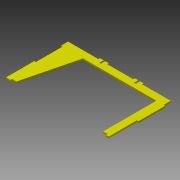
# Autodesk Inventor part: frontLeg
Saved by Autodesk Inventor 2015 SP1 (Build 190203100, 203)
## iProperties
Created: 2015-04-09
Part Number: frontLeg
Material: Generic
Document SubType Name: Modeling
Designer: Iain
Density: 1 g/cm^3
Appearance: Smooth - Yellow
Author: Iain
Autodesk Inventor part; units mm, degrees
sketch "Sketch1" plane through (0, 0, 0) normal (0, 0, 1) x (1, 0, 0)
  line L0 (-590, 351) -> (590, 351)
  line L1 (590, 351) -> (590, -351)
  line L2 (590, -351) -> (-590, -351)
  line L3 (-590, -351) -> (-590, 351)
  point P0 (0, 0)
  point P1 (590, 0)
  point P2 (0, 351)
  dimension "d0" = 1180
  dimension "d1" = 702
  constraints: 8 end point, 2 midpoint, 2 parallel, 1 horizontal, 1 horizontal alignment, 1 perpendicular, 1 vertical alignment
  measures "d0" distance of L0.start L0.end
  measures "d1" distance of L2.end L0.start
extrude "Extrusion1" add sketch "Sketch1" along normal blind 18
sketch "Sketch2" plane through (0, 0, 18) normal (0, 0, 1) x (1, 0, 0)
  line L0 (590, 351) -> (-590, 351) projected
  line L1 (-590, 351) -> (-590, -351) projected
  line L2 (-590, -351) -> (590, -351) projected
  line L3 (590, -351) -> (590, 351) projected
  line L4 (-590, -351) -> (-490, -351) construction
  line L5 (-590, 351) -> (-590, -351) construction
  line L6 (590, 351) -> (-590, 351) construction
  line L7 (0, 351) -> (0, -351) construction
  line L8 (590, -351) -> (490, -351) construction
  line L9 (-590, 271) -> (590, 271) construction
  line L10 (-590, 271) -> (-340, 271) construction
  line L11 (-340, 271) -> (490, 271)
  line L12 (490, 271) -> (490, -351)
  line L13 (490, -351) -> (-490, -351)
  line L14 (-490, -351) -> (-490, -333)
  line L15 (-490, -333) -> (-340, 271)
  point P0 (0, 0)
  point P1 (-590, 0)
  point P2 (-590, 0)
  point P3 (-540, -351)
  point P4 (540, -351)
  point P5 (-590, 0)
  point P6 (590, 0)
  point P7 (-590, 0)
  point P8 (-465, 271)
  point P9 (0, 271)
  dimension "d4" = 100
  dimension "d5" = 80
  dimension "d6" = 250
  dimension "d97" = 18
  constraints: 20 end point, 10 midpoint, 4 symmetric about line, 4 vertical alignment, 3 horizontal, 3 perpendicular, 2 horizontal alignment, 1 collinear, 1 point on line
  measures "d4" distance of L4.start L4.end
  measures "d5" distance between parallel lines of L0 L9
  measures "d6" distance of L10.start L10.end
  measures "d97" distance of L4.end L14.end
extrude "Extrusion2" cut sketch "Sketch2" against normal blind 18 contours L2 L14 L15 L11 L12
sketch "Sketch3" plane through (0, 0, 18) normal (0, 0, 1) x (1, 0, 0)
  line L0 (-340, 271) -> (490, 271) projected
  line L1 (490, 271) -> (490, -351) projected
  line L2 (490, -351) -> (590, -351) projected
  line L3 (590, -351) -> (590, 351) projected
  line L4 (590, 351) -> (-590, 351) projected
  line L5 (-590, 351) -> (-590, -351) projected
  line L6 (-540, -333) -> (540, -333)
  line L7 (540, -333) -> (540, -351)
  line L8 (540, -351) -> (-540, -351)
  line L9 (-540, -351) -> (-540, -333)
  line L10 (490, -351) -> (590, -351) projected
  line L11 (-590, -351) -> (590, -351) projected
  line L12 (-590, -351) -> (-490, -351) projected
  line L13 (-490, -351) -> (-490, -333) projected
  line L14 (-490, -333) -> (-340, 271) projected
  point P0 (0, 0)
  point P1 (540, -351)
  point P2 (0, -351)
  point P3 (-540, -351)
  point P4 (540, -342)
  point P5 (540, -351)
  point P6 (-540, -342)
  point P7 (-540, -351)
  dimension "d10" = 18
  constraints: 8 end point, 5 midpoint, 2 parallel, 2 vertical alignment, 1 horizontal, 1 horizontal alignment, 1 perpendicular, 1 point on line
  measures "d10" distance of L6.end L7.end
extrude "Extrusion3" cut sketch "Sketch3" against normal blind 18 contours L13 L8 L9 L6 | L6 L1 L8 L13 | L6 L7 L2 L1
sketch "Sketch4" plane through (0, 0, 18) normal (0, 0, 1) x (1, 0, 0)
  line L0 (540, -333) -> (540, -351) projected
  line L1 (540, -351) -> (590, -351) projected
  line L2 (590, -351) -> (590, 351) projected
  line L3 (590, 351) -> (-590, 351) projected
  line L4 (-590, 351) -> (-590, -351) projected
  line L5 (-590, -351) -> (-540, -351) projected
  line L6 (-540, -351) -> (-540, -333) projected
  line L7 (-540, -333) -> (-490, -333) projected
  line L8 (-340, 271) -> (490, 271) projected
  line L9 (490, 271) -> (490, -333) projected
  line L10 (490, -333) -> (540, -333) projected
  line L11 (590, -31) -> (572, -31)
  line L12 (572, -31) -> (572, -351)
  line L13 (572, -351) -> (590, -351)
  line L14 (590, -351) -> (590, -31)
  line L15 (-490, -333) -> (-340, 271) projected
  point P0 (0, 0)
  point P1 (581, -351)
  point P2 (565, -351)
  point P3 (590, -191)
  point P4 (590, 0)
  point P5 (581, -31)
  point P6 (490, -31)
  dimension "d13" = 18
  constraints: 8 end point, 6 midpoint, 2 horizontal alignment, 2 parallel, 1 horizontal, 1 perpendicular, 1 vertical alignment
  measures "d13" distance of L11.start L11.end
extrude "Extrusion4" cut sketch "Sketch4" against normal blind 18 contours L12 L11 L2 L1
sketch "Sketch5" plane through (0, 0, 18) normal (0, 0, 1) x (1, 0, 0)
  line L0 (-590, 271) -> (-572, 271)
  line L1 (-572, 271) -> (-572, -31)
  line L2 (-572, -31) -> (-590, -31)
  line L3 (-590, -31) -> (-590, 271)
  line L4 (572, -31) -> (590, -31) projected
  line L5 (590, -31) -> (590, 351) projected
  line L6 (590, 351) -> (-590, 351) projected
  line L7 (-590, 351) -> (-590, -351) projected
  line L8 (-590, -351) -> (-540, -351) projected
  line L9 (-540, -351) -> (-540, -333) projected
  line L10 (-540, -333) -> (-490, -333) projected
  line L11 (-340, 271) -> (490, 271) projected
  line L12 (490, 271) -> (490, -333) projected
  line L13 (490, -333) -> (540, -333) projected
  line L14 (540, -333) -> (540, -351) projected
  line L15 (540, -351) -> (572, -351) projected
  line L16 (572, -351) -> (572, -31) projected
  line L17 (-490, -333) -> (-340, 271) projected
  point P0 (0, 0)
  point P1 (-581, -31)
  point P2 (581, -31)
  point P3 (-581, 271)
  point P4 (75, 271)
  point P5 (-590, 120)
  point P6 (-590, 0)
  dimension "d16" = 18
  constraints: 8 end point, 6 midpoint, 2 horizontal alignment, 2 parallel, 1 horizontal, 1 perpendicular, 1 vertical alignment
  measures "d16" distance of L0.start L0.end
extrude "Extrusion5" cut sketch "Sketch5" against normal blind 18 contours L0 L1 L2 L3
sketch "Sketch6" plane through (0, 0, 18) normal (0, 0, 1) x (1, 0, 0)
  line L0 (-590, 271) -> (-572, 271) projected
  line L1 (-572, 271) -> (-572, -31) projected
  line L2 (-572, -31) -> (-590, -31) projected
  line L3 (-590, -31) -> (-590, -351) projected
  line L4 (-590, -351) -> (-540, -351) projected
  line L5 (-540, -351) -> (-540, -333) projected
  line L6 (-540, -333) -> (-490, -333) projected
  line L7 (-340, 271) -> (490, 271) projected
  line L8 (490, 271) -> (490, -333) projected
  line L9 (490, -333) -> (540, -333) projected
  line L10 (540, -333) -> (540, -351) projected
  line L11 (540, -351) -> (572, -351) projected
  line L12 (572, -351) -> (572, -31) projected
  line L13 (572, -31) -> (590, -31) projected
  line L14 (590, -31) -> (590, 351) projected
  line L15 (590, 351) -> (-590, 351) projected
  line L16 (-590, 351) -> (-590, 271) projected
  line L17 (590, 351) -> (572, 351)
  line L18 (572, 351) -> (572, 271)
  line L19 (572, 271) -> (590, 271)
  line L20 (590, 271) -> (590, 351)
  line L21 (-490, -333) -> (-340, 271) projected
  point P0 (0, 0)
  point P1 (581, 351)
  point P2 (0, 351)
  point P3 (581, 271)
  point P4 (75, 271)
  point P5 (590, 311)
  point P6 (590, 160)
  dimension "d19" = 18
  constraints: 8 end point, 6 midpoint, 2 horizontal alignment, 2 parallel, 1 horizontal, 1 perpendicular, 1 vertical alignment
  measures "d19" distance of L17.start L17.end
extrude "Extrusion6" cut sketch "Sketch6" against normal blind 18 contours L15 L14 L19 L18
fillet "Fillet1" radius 3.175 2 edges at (-340, 271, 9) (490, 271, 9)
sketch "Sketch7" plane through (0, 0, 18) normal (0, 0, 1) x (1, 0, 0)
  line L0 (-246.6667, 369) -> (-146.6667, 369)
  line L1 (-146.6667, 369) -> (-146.6667, 351)
  line L2 (-146.6667, 351) -> (-246.6667, 351)
  line L3 (-246.6667, 351) -> (-246.6667, 369)
  line L4 (590, 271) -> (572, 271) projected
  line L5 (572, 271) -> (572, 351) projected
  line L6 (572, 351) -> (-590, 351) projected
  line L7 (-590, 351) -> (-590, 271) projected
  line L8 (-590, 271) -> (-572, 271) projected
  line L9 (-572, 271) -> (-572, -31) projected
  line L10 (-572, -31) -> (-590, -31) projected
  line L11 (-590, -31) -> (-590, -351) projected
  line L12 (-590, -351) -> (-540, -351) projected
  line L13 (-540, -351) -> (-540, -333) projected
  line L14 (-540, -333) -> (-490, -333) projected
  arc A0 (-337.517, 271) -> (-340.5984, 268.5902) centre (-337.517, 267.825) ccw projected
  line L15 (-337.517, 271) -> (486.825, 271) projected
  arc A1 (490, 267.825) -> (486.825, 271) centre (486.825, 267.825) ccw projected
  line L16 (490, 267.825) -> (490, -333) projected
  line L17 (490, -333) -> (540, -333) projected
  line L18 (540, -333) -> (540, -351) projected
  line L19 (540, -351) -> (572, -351) projected
  line L20 (572, -351) -> (572, -31) projected
  line L21 (572, -31) -> (590, -31) projected
  line L22 (590, -31) -> (590, 271) projected
  line L23 (-490, -333) -> (-340.5984, 268.5902) projected
  point P0 (0, 0)
  point P1 (-196.6667, 351)
  point P2 (-9, 351)
  dimension "d23" = 18
  dimension "d24" = 100
  dimension "d25" = 393.3333
  constraints: 8 end point, 2 midpoint, 2 parallel, 1 horizontal, 1 horizontal alignment, 1 perpendicular
  measures "d23" distance of L0.end L1.end
  measures "d24" distance of L0.start L0.end
  measures "d25" distance of L6.end point (-196.667, 351)
extrude "Extrusion7" add sketch "Sketch7" against normal blind 18 contours L0 L1 L2 L3
ref_plane "Work Plane1" through (0, 351, 0) normal (-1, 0, 0) x (0, 0, 1)
mirror "Mirror1" about plane through (0, 351, 0) normal (-1, 0, 0) of "Extrusion7"
sketch "Sketch8" plane through (0, 0, 18) normal (0, 0, 1) x (1, 0, 0)
  line L0 (590, 271) -> (572, 271) projected
  line L1 (572, 271) -> (572, 351) projected
  line L2 (572, 351) -> (246.6667, 351) projected
  line L3 (246.6667, 351) -> (246.6667, 369) projected
  line L4 (246.6667, 369) -> (146.6667, 369) projected
  line L5 (146.6667, 369) -> (146.6667, 351) projected
  line L6 (146.6667, 351) -> (-146.6667, 351) projected
  line L7 (-146.6667, 369) -> (-146.6667, 351) projected
  line L8 (-246.6667, 369) -> (-146.6667, 369) projected
  line L9 (-246.6667, 351) -> (-246.6667, 369) projected
  line L10 (-246.6667, 351) -> (-590, 351) projected
  line L11 (-590, 351) -> (-590, 271) projected
  line L12 (-590, 271) -> (-572, 271) projected
  line L13 (-572, 271) -> (-572, -31) projected
  line L14 (-572, -31) -> (-590, -31) projected
  line L15 (-590, -31) -> (-590, -351) projected
  line L16 (-590, -351) -> (-540, -351) projected
  line L17 (-540, -351) -> (-540, -333) projected
  line L18 (-540, -333) -> (-490, -333) projected
  arc A0 (-337.517, 271) -> (-340.5984, 268.5902) centre (-337.517, 267.825) ccw projected
  line L19 (-337.517, 271) -> (486.825, 271) projected
  arc A1 (490, 267.825) -> (486.825, 271) centre (486.825, 267.825) ccw projected
  line L20 (490, 267.825) -> (490, -333) projected
  line L21 (490, -333) -> (540, -333) projected
  line L22 (540, -333) -> (540, -351) projected
  line L23 (540, -351) -> (572, -351) projected
  line L24 (572, -351) -> (572, -31) projected
  line L25 (572, -31) -> (590, -31) projected
  line L26 (590, -31) -> (590, 271) projected
  line L27 (-205.6667, 369) -> (-187.6667, 369)
  line L28 (-187.6667, 369) -> (-187.6667, 320)
  line L29 (-187.6667, 320) -> (-205.6667, 320)
  line L30 (-205.6667, 320) -> (-205.6667, 369)
  line L31 (-246.6667, 369) -> (-146.6667, 369) projected
  line L32 (486.825, 271) -> (-337.517, 271) construction
  line L33 (-490, -333) -> (-340.5984, 268.5902) projected
  point P0 (0, 0)
  point P1 (-196.6667, 369)
  point P2 (-196.6667, 369)
  point P3 (-196.6667, 369)
  point P4 (-196.6667, 320)
  point P5 (-590, 311)
  point P6 (-246.6667, 320)
  dimension "d28" = 18
  dimension "d31" = 49
  constraints: 8 end point, 5 midpoint, 2 coincident, 2 parallel, 1 horizontal, 1 horizontal alignment, 1 perpendicular
  measures "d28" distance of L27.start L27.end
  measures "d31" distance of L27.end L28.end
extrude "Extrusion8" cut sketch "Sketch8" against normal blind 18 contours L28 L29 L30 L8
mirror "Mirror2" about plane through (0, 351, 0) normal (-1, 0, 0) of "Extrusion8"
sketch "Sketch9" plane through (0, 0, 18) normal (0, 0, 1) x (1, 0, 0)
  line L0 (187.6667, 320) -> (187.6667, 369) projected
  line L1 (187.6667, 369) -> (146.6667, 369) projected
  line L2 (146.6667, 369) -> (146.6667, 351) projected
  line L3 (146.6667, 351) -> (-146.6667, 351) projected
  line L4 (-146.6667, 369) -> (-146.6667, 351) projected
  line L5 (-187.6667, 369) -> (-146.6667, 369) projected
  line L6 (-187.6667, 369) -> (-187.6667, 320) projected
  line L7 (-187.6667, 320) -> (-205.6667, 320) projected
  line L8 (-205.6667, 320) -> (-205.6667, 369) projected
  line L9 (-246.6667, 369) -> (-205.6667, 369) projected
  line L10 (-246.6667, 351) -> (-246.6667, 369) projected
  line L11 (-246.6667, 351) -> (-590, 351) projected
  line L12 (-590, 351) -> (-590, 271) projected
  line L13 (-590, 271) -> (-572, 271) projected
  line L14 (-572, 271) -> (-572, -31) projected
  line L15 (-572, -31) -> (-590, -31) projected
  line L16 (-590, -31) -> (-590, -351) projected
  line L17 (-590, -351) -> (-540, -351) projected
  line L18 (-540, -351) -> (-540, -333) projected
  line L19 (-540, -333) -> (-490, -333) projected
  arc A0 (-337.517, 271) -> (-340.5984, 268.5902) centre (-337.517, 267.825) ccw projected
  line L20 (-337.517, 271) -> (486.825, 271) projected
  arc A1 (490, 267.825) -> (486.825, 271) centre (486.825, 267.825) ccw projected
  line L21 (490, 267.825) -> (490, -333) projected
  line L22 (490, -333) -> (540, -333) projected
  line L23 (540, -333) -> (540, -351) projected
  line L24 (540, -351) -> (572, -351) projected
  line L25 (572, -351) -> (572, -31) projected
  line L26 (572, -31) -> (590, -31) projected
  line L27 (590, -31) -> (590, 271) projected
  line L28 (590, 271) -> (572, 271) projected
  line L29 (572, 271) -> (572, 351) projected
  line L30 (572, 351) -> (246.6667, 351) projected
  line L31 (246.6667, 351) -> (246.6667, 369) projected
  line L32 (246.6667, 369) -> (205.6667, 369) projected
  line L33 (205.6667, 369) -> (205.6667, 320) projected
  line L34 (205.6667, 320) -> (187.6667, 320) projected
  line L35 (-490, -333) -> (-340.5984, 268.5902) projected
  point P0 (0, 0)
  point P1 (-581, 311)
  point P2 (-590, 311)
  dimension "d32" = 9
  constraints: 1 horizontal alignment, 1 midpoint
  measures "d32" distance of point (-590, 311) point (-581, 311)
hole "Hole1" at (-581, 311, 18) direction (0, 0, -1) diameter 6.35 end through all
sketch "Sketch10" plane through (0, 0, 18) normal (0, 0, 1) x (1, 0, 0)
  circle A0 centre (-581, 311) radius 3.175 projected
  line L0 (187.6667, 320) -> (187.6667, 369) projected
  line L1 (187.6667, 369) -> (146.6667, 369) projected
  line L2 (146.6667, 369) -> (146.6667, 351) projected
  line L3 (146.6667, 351) -> (-146.6667, 351) projected
  line L4 (-146.6667, 369) -> (-146.6667, 351) projected
  line L5 (-187.6667, 369) -> (-146.6667, 369) projected
  line L6 (-187.6667, 369) -> (-187.6667, 320) projected
  line L7 (-187.6667, 320) -> (-205.6667, 320) projected
  line L8 (-205.6667, 320) -> (-205.6667, 369) projected
  line L9 (-246.6667, 369) -> (-205.6667, 369) projected
  line L10 (-246.6667, 351) -> (-246.6667, 369) projected
  line L11 (-246.6667, 351) -> (-590, 351) projected
  line L12 (-590, 351) -> (-590, 271) projected
  line L13 (-590, 271) -> (-572, 271) projected
  line L14 (-572, 271) -> (-572, -31) projected
  line L15 (-572, -31) -> (-590, -31) projected
  line L16 (-590, -31) -> (-590, -351) projected
  line L17 (-590, -351) -> (-540, -351) projected
  line L18 (-540, -351) -> (-540, -333) projected
  line L19 (-540, -333) -> (-490, -333) projected
  arc A1 (-337.517, 271) -> (-340.5984, 268.5902) centre (-337.517, 267.825) ccw projected
  line L20 (-337.517, 271) -> (486.825, 271) projected
  arc A2 (490, 267.825) -> (486.825, 271) centre (486.825, 267.825) ccw projected
  line L21 (490, 267.825) -> (490, -333) projected
  line L22 (490, -333) -> (540, -333) projected
  line L23 (540, -333) -> (540, -351) projected
  line L24 (540, -351) -> (572, -351) projected
  line L25 (572, -351) -> (572, -31) projected
  line L26 (572, -31) -> (590, -31) projected
  line L27 (590, -31) -> (590, 271) projected
  line L28 (590, 271) -> (572, 271) projected
  line L29 (572, 271) -> (572, 351) projected
  line L30 (572, 351) -> (246.6667, 351) projected
  line L31 (246.6667, 351) -> (246.6667, 369) projected
  line L32 (246.6667, 369) -> (205.6667, 369) projected
  line L33 (205.6667, 369) -> (205.6667, 320) projected
  line L34 (205.6667, 320) -> (187.6667, 320) projected
  line L35 (-581, -31) -> (-581, -333) construction
  line L36 (-490, -333) -> (-340.5984, 268.5902) projected
  point P0 (0, 0)
  point P1 (-581, -31)
  point P2 (-515, -333)
  point P3 (-581, -182)
  dimension "d40" = 9
  constraints: 3 midpoint, 2 end point, 1 coincident, 1 horizontal alignment, 1 vertical
  measures "d40" distance of L15.end L35.start
hole "Hole2" at (-581, -182, 18) direction (0, 0, -1) diameter 6.35 end through all
sketch "Sketch11" plane through (0, 0, 18) normal (0, 0, 1) x (1, 0, 0)
  circle A0 centre (-581, -182) radius 3.175 projected
  circle A1 centre (-581, 311) radius 3.175 projected
  line L0 (187.6667, 320) -> (187.6667, 369) projected
  line L1 (187.6667, 369) -> (146.6667, 369) projected
  line L2 (146.6667, 369) -> (146.6667, 351) projected
  line L3 (146.6667, 351) -> (-146.6667, 351) projected
  line L4 (-146.6667, 369) -> (-146.6667, 351) projected
  line L5 (-187.6667, 369) -> (-146.6667, 369) projected
  line L6 (-187.6667, 369) -> (-187.6667, 320) projected
  line L7 (-187.6667, 320) -> (-205.6667, 320) projected
  line L8 (-205.6667, 320) -> (-205.6667, 369) projected
  line L9 (-246.6667, 369) -> (-205.6667, 369) projected
  line L10 (-246.6667, 351) -> (-246.6667, 369) projected
  line L11 (-246.6667, 351) -> (-590, 351) projected
  line L12 (-590, 351) -> (-590, 271) projected
  line L13 (-590, 271) -> (-572, 271) projected
  line L14 (-572, 271) -> (-572, -31) projected
  line L15 (-572, -31) -> (-590, -31) projected
  line L16 (-590, -31) -> (-590, -351) projected
  line L17 (-590, -351) -> (-540, -351) projected
  line L18 (-540, -351) -> (-540, -333) projected
  line L19 (-540, -333) -> (-490, -333) projected
  arc A2 (-337.517, 271) -> (-340.5984, 268.5902) centre (-337.517, 267.825) ccw projected
  line L20 (-337.517, 271) -> (486.825, 271) projected
  arc A3 (490, 267.825) -> (486.825, 271) centre (486.825, 267.825) ccw projected
  line L21 (490, 267.825) -> (490, -333) projected
  line L22 (490, -333) -> (540, -333) projected
  line L23 (540, -333) -> (540, -351) projected
  line L24 (540, -351) -> (572, -351) projected
  line L25 (572, -351) -> (572, -31) projected
  line L26 (572, -31) -> (590, -31) projected
  line L27 (590, -31) -> (590, 271) projected
  line L28 (590, 271) -> (572, 271) projected
  line L29 (572, 271) -> (572, 351) projected
  line L30 (572, 351) -> (246.6667, 351) projected
  line L31 (246.6667, 351) -> (246.6667, 369) projected
  line L32 (246.6667, 369) -> (205.6667, 369) projected
  line L33 (205.6667, 369) -> (205.6667, 320) projected
  line L34 (205.6667, 320) -> (187.6667, 320) projected
  line L35 (-490, -333) -> (-340.5984, 268.5902) projected
  point P0 (0, 0)
  point P1 (581, 120)
  point P2 (590, 120)
  dimension "d48" = 9
  constraints: 1 horizontal alignment, 1 midpoint
  measures "d48" distance of point (590, 120) point (581, 120)
hole "Hole3" at (581, 120, 18) direction (0, 0, -1) diameter 6.35 end through all
sketch "Sketch12" plane through (0, 0, 18) normal (0, 0, 1) x (1, 0, 0)
  circle A0 centre (581, 120) radius 3.175 projected
  circle A1 centre (-581, -182) radius 3.175 projected
  circle A2 centre (-581, 311) radius 3.175 projected
  line L0 (187.6667, 320) -> (187.6667, 369) projected
  line L1 (187.6667, 369) -> (146.6667, 369) projected
  line L2 (146.6667, 369) -> (146.6667, 351) projected
  line L3 (146.6667, 351) -> (-146.6667, 351) projected
  line L4 (-146.6667, 369) -> (-146.6667, 351) projected
  line L5 (-187.6667, 369) -> (-146.6667, 369) projected
  line L6 (-187.6667, 369) -> (-187.6667, 320) projected
  line L7 (-187.6667, 320) -> (-205.6667, 320) projected
  line L8 (-205.6667, 320) -> (-205.6667, 369) projected
  line L9 (-246.6667, 369) -> (-205.6667, 369) projected
  line L10 (-246.6667, 351) -> (-246.6667, 369) projected
  line L11 (-246.6667, 351) -> (-590, 351) projected
  line L12 (-590, 351) -> (-590, 271) projected
  line L13 (-590, 271) -> (-572, 271) projected
  line L14 (-572, 271) -> (-572, -31) projected
  line L15 (-572, -31) -> (-590, -31) projected
  line L16 (-590, -31) -> (-590, -351) projected
  line L17 (-590, -351) -> (-540, -351) projected
  line L18 (-540, -351) -> (-540, -333) projected
  line L19 (-540, -333) -> (-490, -333) projected
  arc A3 (-337.517, 271) -> (-340.5984, 268.5902) centre (-337.517, 267.825) ccw projected
  line L20 (-337.517, 271) -> (486.825, 271) projected
  arc A4 (490, 267.825) -> (486.825, 271) centre (486.825, 267.825) ccw projected
  line L21 (490, 267.825) -> (490, -333) projected
  line L22 (490, -333) -> (540, -333) projected
  line L23 (540, -333) -> (540, -351) projected
  line L24 (540, -351) -> (572, -351) projected
  line L25 (572, -351) -> (572, -31) projected
  line L26 (572, -31) -> (590, -31) projected
  line L27 (590, -31) -> (590, 271) projected
  line L28 (590, 271) -> (572, 271) projected
  line L29 (572, 271) -> (572, 351) projected
  line L30 (572, 351) -> (246.6667, 351) projected
  line L31 (246.6667, 351) -> (246.6667, 369) projected
  line L32 (246.6667, 369) -> (205.6667, 369) projected
  line L33 (205.6667, 369) -> (205.6667, 320) projected
  line L34 (205.6667, 320) -> (187.6667, 320) projected
  line L35 (-196.6667, 320) -> (-196.6667, 271) construction
  line L36 (-187.6667, 320) -> (-205.6667, 320) construction
  line L37 (-490, -333) -> (-340.5984, 268.5902) projected
  point P0 (0, 0)
  point P1 (74.654, 271)
  point P2 (-196.6667, 295.5)
  point P3 (-196.6667, 295.5)
  constraints: 4 midpoint, 2 coincident, 2 end point, 1 horizontal alignment, 1 vertical, 1 vertical alignment
hole "Hole4" at (-196.6667, 295.5, 18) direction (0, 0, -1) diameter 6.35 end through all
mirror "Mirror3" about plane through (0, 351, 0) normal (-1, 0, 0) of "Hole4"
sketch "Sketch13" plane through (0, 0, 18) normal (0, 0, 1) x (1, 0, 0)
  line L0 (-590, 271) -> (-572, 271) projected
  point P0 (0, 0)
  point P1 (-572, 267.825)
  dimension "d63" = 3.175
  constraints: 1 vertical alignment
  measures "d63" distance from line of L0 point (-572, 267.825)
hole "Hole5" at (-572, 267.825, 18) direction (0, 0, -1) diameter 6.35 end through all
ref_plane "Work Plane2" through (-590, 120, 0) normal (0, -1, 0) x (1, 0, 0)
mirror "Mirror4" about plane through (-590, 120, 0) normal (0, -1, 0) of "Hole5"
sketch "Sketch14" plane through (0, 0, 18) normal (0, 0, 1) x (1, 0, 0)
  arc A0 (-572, -31) -> (-572, -24.65) centre (-572, -27.825) ccw projected
  line L0 (-572, -31) -> (-590, -31) projected
  line L1 (-590, -31) -> (-590, -351) projected
  line L2 (-590, -351) -> (-540, -351) projected
  line L3 (-540, -351) -> (-540, -333) projected
  line L4 (-540, -333) -> (-490, -333) projected
  arc A1 (-337.517, 271) -> (-340.5984, 268.5902) centre (-337.517, 267.825) ccw projected
  line L5 (-337.517, 271) -> (486.825, 271) projected
  arc A2 (490, 267.825) -> (486.825, 271) centre (486.825, 267.825) ccw projected
  line L6 (490, 267.825) -> (490, -333) projected
  line L7 (490, -333) -> (540, -333) projected
  line L8 (540, -333) -> (540, -351) projected
  line L9 (540, -351) -> (572, -351) projected
  line L10 (572, -351) -> (572, -31) projected
  line L11 (572, -31) -> (590, -31) projected
  line L12 (590, -31) -> (590, 271) projected
  line L13 (590, 271) -> (572, 271) projected
  line L14 (572, 271) -> (572, 351) projected
  line L15 (572, 351) -> (246.6667, 351) projected
  line L16 (246.6667, 351) -> (246.6667, 369) projected
  line L17 (246.6667, 369) -> (205.6667, 369) projected
  line L18 (205.6667, 369) -> (205.6667, 320) projected
  line L19 (205.6667, 320) -> (187.6667, 320) projected
  line L20 (187.6667, 320) -> (187.6667, 369) projected
  line L21 (187.6667, 369) -> (146.6667, 369) projected
  line L22 (146.6667, 369) -> (146.6667, 351) projected
  line L23 (146.6667, 351) -> (-146.6667, 351) projected
  line L24 (-146.6667, 369) -> (-146.6667, 351) projected
  line L25 (-187.6667, 369) -> (-146.6667, 369) projected
  line L26 (-187.6667, 369) -> (-187.6667, 320) projected
  line L27 (-187.6667, 320) -> (-205.6667, 320) projected
  line L28 (-205.6667, 320) -> (-205.6667, 369) projected
  line L29 (-246.6667, 369) -> (-205.6667, 369) projected
  line L30 (-246.6667, 351) -> (-246.6667, 369) projected
  line L31 (-246.6667, 351) -> (-590, 351) projected
  line L32 (-590, 351) -> (-590, 271) projected
  line L33 (-590, 271) -> (-572, 271) projected
  arc A3 (-572, 264.65) -> (-572, 271) centre (-572, 267.825) ccw projected
  line L34 (-572, 264.65) -> (-572, -24.65) projected
  circle A4 centre (196.6667, 295.5) radius 3.175 projected
  circle A5 centre (-196.6667, 295.5) radius 3.175 projected
  circle A6 centre (581, 120) radius 3.175 projected
  circle A7 centre (-581, -182) radius 3.175 projected
  circle A8 centre (-581, 311) radius 3.175 projected
  line L35 (-490, -333) -> (-340.5984, 268.5902) projected
  point P0 (0, 0)
  point P1 (572, 274.175)
  dimension "d71" = 3.175
  constraints: 1 vertical alignment
  measures "d71" distance from line of L13 point (572, 274.175)
hole "Hole6" at (572, 274.175, 18) direction (0, 0, -1) diameter 6.35 end through all
mirror "Mirror5" about plane through (-590, 120, 0) normal (0, -1, 0) of "Hole6"
sketch "Sketch15" plane through (0, 0, 18) normal (0, 0, 1) x (1, 0, 0)
  line L0 (-540, -351) -> (-540, -333) projected
  line L1 (-540, -333) -> (-490, -333) projected
  point P0 (0, 0)
  point P1 (-536.825, -333)
  point P2 (-515, -333)
  point P3 (-485.6592, -333)
  dimension "d79" = 3.175
  constraints: 1 horizontal alignment, 1 midpoint
  measures "d79" distance from line of L0 point (-536.825, -333)
hole "Hole7" at (-536.825, -333, 18) direction (0, 0, -1) diameter 6.35 end through all
mirror "Mirror6" about plane through (0, 351, 0) normal (-1, 0, 0) of "Hole7"
sketch "Sketch16" plane through (0, 0, 18) normal (0, 0, 1) x (1, 0, 0)
  arc A0 (540, -333) -> (533.65, -333) centre (536.825, -333) ccw projected
  line L0 (540, -333) -> (540, -351) projected
  line L1 (540, -351) -> (572, -351) projected
  line L2 (572, -351) -> (572, -37.35) projected
  arc A1 (572, -31) -> (572, -37.35) centre (572, -34.175) ccw projected
  line L3 (572, -31) -> (590, -31) projected
  line L4 (590, -31) -> (590, 271) projected
  line L5 (590, 271) -> (572, 271) projected
  arc A2 (572, 277.35) -> (572, 271) centre (572, 274.175) ccw projected
  line L6 (572, 277.35) -> (572, 351) projected
  line L7 (572, 351) -> (246.6667, 351) projected
  line L8 (246.6667, 351) -> (246.6667, 369) projected
  line L9 (246.6667, 369) -> (205.6667, 369) projected
  line L10 (205.6667, 369) -> (205.6667, 320) projected
  line L11 (205.6667, 320) -> (187.6667, 320) projected
  line L12 (187.6667, 320) -> (187.6667, 369) projected
  line L13 (187.6667, 369) -> (146.6667, 369) projected
  line L14 (146.6667, 369) -> (146.6667, 351) projected
  line L15 (146.6667, 351) -> (-146.6667, 351) projected
  line L16 (-146.6667, 369) -> (-146.6667, 351) projected
  line L17 (-187.6667, 369) -> (-146.6667, 369) projected
  line L18 (-187.6667, 369) -> (-187.6667, 320) projected
  line L19 (-187.6667, 320) -> (-205.6667, 320) projected
  line L20 (-205.6667, 320) -> (-205.6667, 369) projected
  line L21 (-246.6667, 369) -> (-205.6667, 369) projected
  line L22 (-246.6667, 351) -> (-246.6667, 369) projected
  line L23 (-246.6667, 351) -> (-590, 351) projected
  line L24 (-590, 351) -> (-590, 271) projected
  line L25 (-590, 271) -> (-572, 271) projected
  arc A3 (-572, 264.65) -> (-572, 271) centre (-572, 267.825) ccw projected
  line L26 (-572, 264.65) -> (-572, -24.65) projected
  arc A4 (-572, -31) -> (-572, -24.65) centre (-572, -27.825) ccw projected
  line L27 (-572, -31) -> (-590, -31) projected
  line L28 (-590, -31) -> (-590, -351) projected
  line L29 (-590, -351) -> (-540, -351) projected
  line L30 (-540, -351) -> (-540, -333) projected
  arc A5 (-533.65, -333) -> (-540, -333) centre (-536.825, -333) ccw projected
  line L31 (-533.65, -333) -> (-490, -333) projected
  arc A6 (-337.517, 271) -> (-340.5984, 268.5902) centre (-337.517, 267.825) ccw projected
  line L32 (-337.517, 271) -> (486.825, 271) projected
  arc A7 (490, 267.825) -> (486.825, 271) centre (486.825, 267.825) ccw projected
  line L33 (490, 267.825) -> (490, -333) projected
  line L34 (490, -333) -> (533.65, -333) projected
  circle A8 centre (196.6667, 295.5) radius 3.175 projected
  circle A9 centre (-196.6667, 295.5) radius 3.175 projected
  circle A10 centre (581, 120) radius 3.175 projected
  circle A11 centre (-581, -182) radius 3.175 projected
  circle A12 centre (-581, 311) radius 3.175 projected
  line L35 (-490, -333) -> (-340.5984, 268.5902) projected
  point P0 (0, 0)
  point P1 (-249.8417, 351)
  point P2 (-205.6667, 323.175)
  dimension "d87" = 3.175
  dimension "d88" = 3.175
  constraints: 1 horizontal alignment, 1 vertical alignment
  measures "d87" horizontal distance of L21.start point (-249.842, 351)
  measures "d88" distance from line of L19 point (-205.667, 323.175)
hole "Hole8" at (-249.8417, 351, 18) at (-205.6667, 323.175, 18) direction (0, 0, -1) diameter 6.35 end through all
ref_plane "Work Plane3" through (-196.6667, 320, 18) normal (-1, 0, 0) x (0, 0, 1)
mirror "Mirror7" about plane through (-196.6667, 320, 18) normal (-1, 0, 0) of "Hole8"
mirror "Mirror8" about plane through (0, 351, 0) normal (-1, 0, 0) of "Hole8", "Mirror7"
equation "\"d0\" = tableLength"
equation "\"d1\" = legHeight"
equation "\"d2\" = PlyThickness"
equation "\"d4\" = legBaseWidth"
equation "\"d5\" = legTopDepth"
equation "\"d6\" = legTopWidthLong"
equation "\"d97\" = plyThickness"
equation "\"d7\" = PlyThickness"
equation "\"d10\" = PlyThickness"
equation "\"d11\" = PlyThickness"
equation "\"d13\" = PlyThickness"
equation "\"d14\" = PlyThickness"
equation "\"d16\" = PlyThickness"
equation "\"d17\" = PlyThickness"
equation "\"d19\" = PlyThickness"
equation "\"d20\" = PlyThickness"
equation "\"d22\" = 0.5 * millDiameter"
equation "\"d23\" = legTopTabHeight"
equation "\"d24\" = legTabTotalWidth"
equation "\"d25\" = 0.333333 * tableLength"
equation "\"d26\" = PlyThickness"
equation "\"d28\" = plyThickness"
equation "\"d31\" = legTopSlotDepth"
equation "\"d29\" = PlyThickness"
equation "\"d32\" = 0.5 * plyThickness"
equation "\"d33\" = millDiameter"
equation "\"d40\" = 0.5 * plyThickness"
equation "\"d41\" = millDiameter"
equation "\"d48\" = 0.5 * plyThickness"
equation "\"d49\" = millDiameter"
equation "\"d56\" = millDiameter"
equation "\"d63\" = 0.5 * millDiameter"
equation "\"d64\" = millDiameter"
equation "\"d71\" = 0.5 * millDiameter"
equation "\"d72\" = millDiameter"
equation "\"d79\" = 0.5 * millDiameter"
equation "\"d80\" = millDiameter"
equation "\"d87\" = 0.5 * millDiameter"
equation "\"d88\" = 0.5 * millDiameter"
equation "\"d89\" = millDiameter"
equation "\"PlyThickness\" = 18"
equation "\"legHeight\" = 702"
equation "\"plyThickness\" = 18"
equation "\"tableLength\" = 1180"
equation "\"legTopWidthLong\" = 250"
equation "\"legBaseWidth\" = 100"
equation "\"legTopDepth\" = 80"
equation "\"millDiameter\" = 6.35"
equation "\"legTopTabHeight\" = 18"
equation "\"legTabTotalWidth\" = 100"
equation "\"legTopSlotDepth\" = 49"
body "Solid1"
